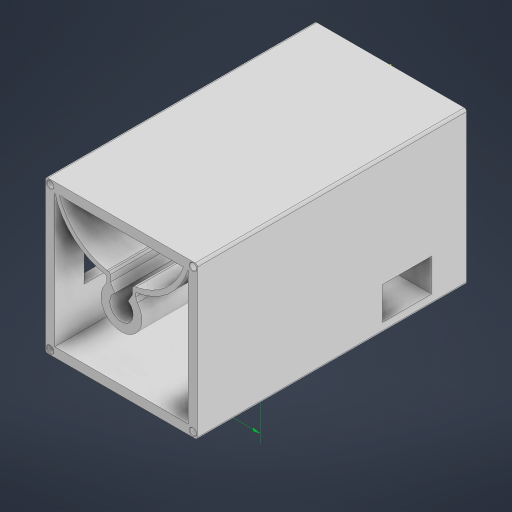
# Autodesk Inventor part: doser-housing
Saved by Autodesk Inventor 2023 (Build 270158000, 158)
## iProperties
Created: 2022-11-09
Part Number: doser-housing
Material: Generic
Document SubType Name: Modeling
Designer: Mike
Density: 1 g/cm^3
Appearance: Default
Author: Mike
Autodesk Inventor part; units mm, degrees
ref_plane "YZ Plane" through (0, 0, 0) normal (1, 0, 0) x (0, 1, 0)
ref_plane "XZ Plane" through (0, 0, 0) normal (0, 1, 0) x (-1, 0, 0)
ref_plane "XY Plane" through (0, 0, 0) normal (0, 0, 1) x (1, 0, 0)
sketch "Sketch1" plane through (0, 0, 0) normal (0, 0, 1) x (1, 0, 0)
  circle A0 centre (0, 0) radius 5
  line L0 (15.5, -15.5) -> (-15.5, -15.5) construction
  line L1 (-15.5, -15.5) -> (-15.5, 15.5) construction
  line L2 (-15.5, 15.5) -> (15.5, 15.5) construction
  line L3 (15.5, 15.5) -> (15.5, -15.5) construction
  line L4 (15.5, -15.5) -> (-15.5, 15.5) construction
  line L5 (-15.5, -15.5) -> (15.5, 15.5) construction
  circle A1 centre (-15.5, 15.5) radius 1.5
  circle A2 centre (15.5, 15.5) radius 1.5
  circle A3 centre (15.5, -15.5) radius 1.5
  circle A4 centre (-15.5, -15.5) radius 1.5
  line L6 (31.5, -32.5) -> (-31.5, -32.5)
  line L7 (-32.5, -31.5) -> (-32.5, 31.5)
  line L8 (-31.5, 32.5) -> (31.5, 32.5)
  line L9 (32.5, 31.5) -> (32.5, -31.5)
  line L10 (32.5, -32.5) -> (-32.5, 32.5) construction
  line L11 (-32.5, -32.5) -> (32.5, 32.5) construction
  arc A5 (-31.5, 32.5) -> (-32.5, 31.5) centre (-31.5, 31.5) ccw
  arc A6 (-32.5, -31.5) -> (-31.5, -32.5) centre (-31.5, -31.5) ccw
  arc A7 (31.5, -32.5) -> (32.5, -31.5) centre (31.5, -31.5) ccw
  arc A8 (32.5, 31.5) -> (31.5, 32.5) centre (31.5, 31.5) ccw
  arc A9 (-6.8415, 5.4549) -> (6.8415, 5.4549) centre (0, 0) ccw
  line L12 (-6.1872, 7.3252) -> (-6.1872, 8.9372)
  line L13 (-6.1872, 8.9372) -> (6.1872, 8.9372)
  line L14 (6.1872, 8.9372) -> (6.1872, 7.3252)
  arc A10 (-6.8415, 5.4549) -> (-6.1872, 7.3252) centre (-9.1872, 7.3252) ccw
  arc A11 (6.1872, 7.3252) -> (6.8415, 5.4549) centre (9.1872, 7.3252) ccw
  line L15 (28.5, 28.5) -> (-28.5, 28.5)
  line L16 (-28.5, 28.5) -> (-28.5, -28.5)
  line L17 (-28.5, -28.5) -> (28.5, -28.5)
  line L18 (28.5, -28.5) -> (28.5, 28.5)
  point P0 (-6.1872, 6.1872)
  point P1 (6.1872, 6.1872)
  dimension "d0" = 10
  dimension "d1" = 31
  dimension "d2" = 31
  dimension "d3" = 3
  dimension "d4" = 3
  dimension "d5" = 3
  dimension "d6" = 3
  dimension "d7" = 65
  dimension "d8" = 65
  dimension "d9" = 1
  dimension "d10" = 17.5
  dimension "d11" = 2.75
  dimension "d12" = 3
  dimension "d13" = 4
  constraints: 38 end point, 16 point on circle, 12 centre point, 12 point on line, 12 tangent, 6 coincident, 6 parallel, 4 equal radius, 4 midpoint, 4 perpendicular, 2 horizontal, 2 vertical, 3 other
  measures "d0" diameter of A0
  measures "d1" distance of A2.centre A1.centre
  measures "d2" distance of A4.centre A1.centre
  measures "d3" diameter of A1
  measures "d4" diameter of A2
  measures "d5" diameter of A3
  measures "d6" diameter of A4
  measures "d7" distance of L11.start L10.end
  measures "d8" distance of L10.start L11.start
  measures "d9" radius of A5
  measures "d10" diameter of A9
  measures "d11" distance of point (-6.187, 6.187) L12.end
  measures "d12" radius of A10
  measures "d13" distance between parallel lines of L8 L15
extrude "Extrusion1" add sketch "Sketch1" along normal blind 115 contours L6 A6 L7 A5 L8 A8 L9 A7 | A10 L12 L13 L14 A11 A9
extrude "Extrusion2" add sketch "Sketch1" along normal blind 15 contours L18 L17 L16 L15
sketch "Sketch2" plane through (-31.5, 32.5, 0) normal (0, 1, 0) x (1, 0, 0)
  point P0 (31.5, 0)
sketch "Sketch3" plane through (0, 0, 115) normal (0, 0, 1) x (1, 0, 0)
  arc A0 (-28.5, 28.5) -> (-6.1872, 8.9372) centre (-2.0793, 36.1286) ccw
  line L0 (6.1872, 7.3252) -> (6.1872, 8.9372) projected
  line L1 (28.5, 28.5) -> (28.5, -28.5) projected
  arc A1 (6.1872, 8.9372) -> (28.5, 28.5) centre (2.0793, 36.1286) ccw
  line L2 (6.1872, 8.9372) -> (-6.1872, 8.9372) projected
  line L3 (-28.5, 28.5) -> (28.5, 28.5) projected
  line L4 (-28.5, 28.5) -> (-26.5, 28.5)
  line L5 (28.5, 28.5) -> (26.5, 28.5)
  arc A2 (-26.5, 28.5) -> (-6.1872, 10.9372) centre (-1.4006, 37.0013) ccw
  arc A3 (6.1872, 10.9372) -> (26.5, 28.5) centre (1.4006, 37.0013) ccw
  line L6 (-6.1872, 8.9372) -> (-6.1872, 7.3252) projected
  line L7 (-6.1872, 8.9372) -> (-6.1872, 7.3252)
  line L8 (-6.1872, 7.3252) -> (-4.6872, 7.3252)
  line L9 (-4.6872, 7.3252) -> (-4.6872, 10.1872)
  line L10 (6.1872, 8.9372) -> (6.1872, 7.3252)
  line L11 (6.1872, 7.3252) -> (4.6872, 7.3252)
  line L12 (4.6872, 7.3252) -> (4.6872, 10.1872)
  line L13 (-6.1872, 10.9372) -> (-5.4372, 10.9372)
  line L14 (5.4372, 10.9372) -> (6.1872, 10.9372)
  line L15 (-4.6872, 10.1872) -> (-5.4372, 10.9372)
  line L16 (4.6872, 10.1872) -> (5.4372, 10.9372)
  line L17 (-5.4372, 10.9372) -> (5.4372, 10.9372)
  line L18 (4.6872, 7.3252) -> (-4.6872, 7.3252)
  line L19 (-4.6872, 7.3252) -> (-2.8356, 4.1182)
  line L20 (-4.6872, 7.3252) -> (-0.7761, 7.3252) construction
  line L21 (4.6872, 7.1776) -> (8.8154, 7.1776) construction
  circle A4 centre (0, 0) radius 5
  line L22 (4.6872, 7.3252) -> (2.8356, 4.1182)
  line L23 (4.6872, 7.3252) -> (9.2305, 7.3252) construction
  circle A5 centre (0, 0) radius 8.75
  point P0 (-4.6872, 10.9372)
  point P1 (4.6872, 10.9372)
  point P2 (-4.7858, 7.3252)
  point P3 (-4.6872, 7.3887)
  point P4 (4.6872, 7.3887)
  point P5 (4.7858, 7.3252)
  dimension "d18" = 27.5
  dimension "d19" = 27.5
  dimension "d20" = 2
  dimension "d21" = 2
  dimension "d23" = 26.5
  dimension "d24" = 26.5
  dimension "d25" = 22.3128
  dimension "d26" = 29.9006
  dimension "d27" = 1.5
  dimension "d28" = 1.5
  dimension "d29" = 2
  dimension "d30" = 2
  dimension "d31" = 0.75
  dimension "d32" = 0.75
  dimension "d33" = 0.75
  dimension "d34" = 0.75
  dimension "d35" = 60
  dimension "d37" = 120
  dimension "d38" = 10
  dimension "d39" = 17.5
  constraints: 38 end point, 10 point on circle, 7 point on line, 6 centre point, 5 perpendicular, 3 horizontal, 2 coincident, 1 collinear
  measures "d18" radius of A0
  measures "d19" radius of A1
  measures "d20" distance of L3.start L4.end
  measures "d21" distance of L1.start L5.end
  measures "d23" radius of A2
  measures "d24" radius of A3
  measures "d25" distance from line of L14.end L1
  measures "d26" distance from line of A2.centre L1
  measures "d27" distance between parallel lines of L9 L7
  measures "d28" distance between parallel lines of L0 L12
  measures "d29" distance between parallel lines of L2 L14
  measures "d30" distance between parallel lines of L2 L13
  measures "d31" distance of L9.end point (-4.687, 10.937)
  measures "d32" distance of L13.end point (-4.687, 10.937)
  measures "d33" distance of L12.end point (4.687, 10.937)
  measures "d34" distance of L14.start point (4.687, 10.937)
  measures "d35" angle of L19 L20
  measures "d37" angle of L22 L23
  measures "d38" diameter of A4
  measures "d39" diameter of A5
extrude "Extrusion3" add sketch "Sketch3" against normal blind 105 contours L3 A2 L13 L15 L9 L2 A0 | L2 L9 A5 L8 L6 | L3 A1 L2 L12 L16 L14 A3 | L2 L0 L11 A5 L12
extrude "Extrusion4" cut sketch "Sketch3" against normal blind 80 contours L9 L15 L17 L16 L12 L2 | L2 L12 A5 L9 | A5 L12 L18 L9 | L18 L22 A4 L19
extrude "Extrusion5" add sketch "Sketch1" along normal blind 15 contours A1 | A2
chamfer "Chamfer1" distance 2 angle 45 1 edges at (0, 8.9372, 35)
sketch "Sketch4" plane through (0, 0, 115) normal (0, 0, 1) x (1, 0, 0)
  line L0 (30.5, -30.5) -> (-30.5, -30.5) construction
  line L1 (-30.5, -30.5) -> (-30.5, 30.5) construction
  line L2 (-30.5, 30.5) -> (30.5, 30.5) construction
  line L3 (30.5, 30.5) -> (30.5, -30.5) construction
  line L4 (30.5, -30.5) -> (-30.5, 30.5) construction
  line L5 (-30.5, -30.5) -> (30.5, 30.5) construction
  circle A0 centre (-30.5, 30.5) radius 1.45
  circle A1 centre (30.5, 30.5) radius 1.45
  circle A2 centre (30.5, -30.5) radius 1.45
  circle A3 centre (-30.5, -30.5) radius 1.45
  point P0 (0, 0)
  dimension "d52" = 61
  dimension "d53" = 61
  dimension "d54" = 2.9
  dimension "d55" = 2.9
  dimension "d56" = 2.9
  dimension "d57" = 2.9
  constraints: 12 end point, 4 centre point, 4 coincident, 2 midpoint, 2 parallel, 1 horizontal, 1 perpendicular
  measures "d52" distance of L1.end L2.end
  measures "d53" distance of L0.end L1.end
  measures "d54" diameter of A0
  measures "d55" diameter of A1
  measures "d56" diameter of A2
  measures "d57" diameter of A3
extrude "Extrusion6" cut sketch "Sketch4" against normal blind 60
chamfer "Chamfer2" distance 0.2 angle 45 6 edges at (-31.95, 30.5, 115) (29.05, 30.5, 115) (-31.95, -30.5, 115) (-17, -15.5, 15) (14, -15.5, 15) (29.05, -30.5, 115)
sketch "Sketch5" plane through (-32.5, -31.5, 0) normal (-1, 0, 0) x (0, 0, 1)
  line L0 (17.5, 37.5) -> (72.5, 37.5)
  line L1 (72.5, 37.5) -> (72.5, 20)
  line L2 (72.5, 20) -> (17.5, 20)
  line L3 (17.5, 20) -> (17.5, 37.5)
  line L4 (85, 37.5) -> (102.5, 37.5)
  line L5 (102.5, 37.5) -> (102.5, 20)
  line L6 (102.5, 20) -> (85, 20)
  line L7 (85, 20) -> (85, 37.5)
  line L8 (0, 63) -> (0, 0) projected
  line L9 (115, 63) -> (115, 0) projected
  point P0 (0, 31.5)
  dimension "d63" = 12.5
  dimension "d64" = 17.5
  dimension "d65" = 17.5
  dimension "d66" = 55
  dimension "d67" = 12.5
  dimension "d68" = 20
  constraints: 16 end point, 4 parallel, 2 horizontal, 2 perpendicular, 2 point on line
  measures "d63" distance between parallel lines of L7 L1
  measures "d64" distance of L2.end L0.start
  measures "d65" distance between parallel lines of L8 L3
  measures "d66" distance of L1.end L2.end
  measures "d67" distance between parallel lines of L9 L5
  measures "d68" distance from line of L8.end L2
extrude "Extrusion7" cut sketch "Sketch5" against normal up to surface (4 mm away)
sketch "Sketch6" plane through (32.5, -31.5, 0) normal (1, 0, 0) x (0, 0, -1)
  line L0 (-15, 60) -> (-15, 3) projected
  line L1 (-15, 3) -> (-36, 3)
  line L2 (-36, 3) -> (-36, 17)
  line L3 (-36, 17) -> (-15, 17)
  line L4 (-15, 17) -> (-15, 3)
  point P0 (0, 31.5)
  dimension "d71" = 21
  dimension "d72" = 14
  constraints: 8 end point, 2 parallel, 1 horizontal, 1 perpendicular
  measures "d71" distance of L2.end L3.end
  measures "d72" distance of L1.end L2.end
extrude "Extrusion8" cut sketch "Sketch6" against normal up to surface (4 mm away)
equation "\"d5\" = d4"
equation "\"d6\" = d5"
equation "\"d32\" = d31"
equation "\"d33\" = d31"
equation "\"d34\" = d33"
body "Solid1"
